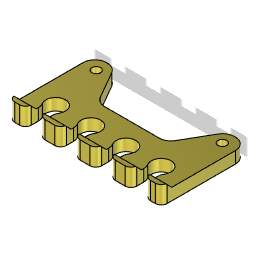
cable_holder (Autodesk Fusion 360 design; units mm, degrees)
Autodesk Fusion 360 part; units mm, degrees
note: some values were not read from the file. Set by a fixed rule: which sketch regions a step uses.
sketch "Sketch1" plane through (0, 0, 0) normal (0, 0, 1) x (1, 0, 0)
  line L0 (0, 0) -> (78, 0)
  line L1 (78, 0) -> (78, 24)
  line L2 (0, 24) -> (0, 0)
  line L3 (12, 12) -> (12, 24) construction
  line L4 (8.5, 15.5707) -> (15.5, 15.5707) construction
  line L5 (8.5, 15.5707) -> (8.5, 24)
  line L6 (15.5, 15.5707) -> (15.5, 24)
  arc A0 (8.5, 15.5707) -> (15.5, 15.5707) centre (12, 12) ccw
  line L7 (8.5, 24) -> (0, 24)
  line L8 (33.5, 15.5707) -> (33.5, 24)
  line L9 (26.5, 15.5707) -> (26.5, 24)
  arc A1 (26.5, 15.5707) -> (33.5, 15.5707) centre (30, 12) ccw
  line L10 (51.5, 15.5707) -> (51.5, 24)
  line L11 (44.5, 15.5707) -> (44.5, 24)
  arc A2 (44.5, 15.5707) -> (51.5, 15.5707) centre (48, 12) ccw
  line L12 (69.5, 15.5707) -> (69.5, 24)
  line L13 (62.5, 15.5707) -> (62.5, 24)
  arc A3 (62.5, 15.5707) -> (69.5, 15.5707) centre (66, 12) ccw
  line L14 (26.5, 24) -> (15.5, 24)
  line L15 (44.5, 24) -> (33.5, 24)
  line L16 (78, 24) -> (69.5, 24)
  line L17 (62.5, 24) -> (51.5, 24)
  dimension "d1" = 10
  dimension "d3" = 12
  dimension "d4" = 12
  dimension "d5" = 3.5
  dimension "d6" = 3.5
  dimension "d7" = 12
  dimension "d10" = 18
  dimension "d11" = 0
  dimension "d12" = 12
  constraint horizontal L0
  constraint vertical L1
  constraint horizontal L16
  constraint vertical L2
  constraint coincident L0.start L2.end
  constraint coincident L3.start A0.centre
  constraint perpendicular L3 L16
  constraint perpendicular L3 L4
  constraint coincident L5.end L16
  constraint perpendicular L4 L5
  constraint perpendicular L6 L16
  constraint collinear L7 L16
  constraint coincident L3.end L16
  constraint collinear L14 L16
  constraint collinear L15 L16
  constraint collinear L16 L17
  measures "d1" diameter of A0
  measures "d3" distance of L3.start L2
  measures "d4" distance of L3.start L0
  measures "d5" distance of L3 L4.end
  measures "d6" distance of L3 L4.start
  measures "d7" distance of L3.start L16
  measures "d12" distance of L1 A3.centre
  measures "d28" angle of L3.start
extrude "Extrude1" add sketch "Sketch1" along normal blind 9
sketch "Sketch2" plane through (0, 0, 0) normal (-1, 0, 0) x (0, -1, 0)
  line L0 (-24, 0) -> (0, 0)
  line L1 (0, 0) -> (0, 9)
  line L2 (0, 9) -> (-24, 9)
  line L3 (-24, 9) -> (-24, 0)
  line L4 (-24, 9) -> (-16.9844, 9) construction
  line L5 (-18.6, 6) -> (0, 6)
  line L6 (-24, 9) -> (0, 9)
  line L7 (0, 6) -> (0, 9)
  line L8 (-24, 9) -> (-21.6, 9)
  line L9 (-18.6, 6) -> (-21.6, 9)
  dimension "d17" = 3
  dimension "d34" = 45
  dimension "d35" = 2.4
  constraint horizontal L4
  constraint coincident L2.end L3.start
  constraint coincident L1 L5.end
  constraint perpendicular L1 L5
  constraint coincident L1.end L2.start
  constraint coincident L4 L8.end
  constraint perpendicular L3 L8
  measures "d17" distance of L2 L5
  measures "d34" angle of L6 L9
  measures "d35" distance of L2.end L8.end
extrude "Extrude2" cut sketch "Sketch2" against normal through all contours L1 L2 L5 L6 L7 L9
sketch "Sketch3" plane through (0, 0, 6) normal (0, 0, 1) x (-1, 0, 0)
  line L0 (-15.5, -18.6) -> (-15.5, -15.5707)
  arc A0 (-8.5, -15.5707) -> (-15.5, -15.5707) centre (-12, -12) ccw
  line L1 (-8.5, -15.5707) -> (-8.5, -18.6)
  line L2 (0, -18.6) -> (0, 0)
  line L3 (0, 0) -> (-78, 0)
  line L4 (-78, 0) -> (-78, -18.6)
  line L5 (-69.5, -18.6) -> (-69.5, -15.5707)
  arc A1 (-62.5, -15.5707) -> (-69.5, -15.5707) centre (-66, -12) ccw
  line L6 (-62.5, -15.5707) -> (-62.5, -18.6)
  line L7 (-51.5, -18.6) -> (-51.5, -15.5707)
  arc A2 (-44.5, -15.5707) -> (-51.5, -15.5707) centre (-48, -12) ccw
  line L8 (-44.5, -15.5707) -> (-44.5, -18.6)
  line L9 (-33.5, -18.6) -> (-33.5, -15.5707)
  arc A3 (-26.5, -15.5707) -> (-33.5, -15.5707) centre (-30, -12) ccw
  line L10 (-26.5, -15.5707) -> (-26.5, -18.6)
  line L11 (0, 0) -> (0, 20)
  line L12 (0, 20) -> (-10, 20)
  line L13 (-10, 20) -> (-21.547, 0)
  line L14 (-78, 0) -> (-78, 20)
  line L15 (-78, 20) -> (-68, 20)
  line L16 (-68, 20) -> (-56.453, 0)
  line L17 (0, 0) -> (-21.547, 0)
  line L18 (-56.453, 0) -> (-78, 0)
  line L19 (-8.5, -18.6) -> (0, -18.6)
  line L20 (-78, -18.6) -> (-69.5, -18.6)
  line L21 (-62.5, -18.6) -> (-51.5, -18.6)
  line L22 (-44.5, -18.6) -> (-33.5, -18.6)
  line L23 (-26.5, -18.6) -> (-15.5, -18.6)
  dimension "d25" = 20
  dimension "d26" = 10
  dimension "d27" = 10
  dimension "d28" = 60
  dimension "d29" = 60
  constraint coincident L2.end L3.start
  constraint perpendicular L3 L11
  constraint perpendicular L11 L12
  constraint coincident L3 L13.end
  constraint coincident L3.end L4.start
  constraint perpendicular L3 L14
  constraint perpendicular L14 L15
  constraint coincident L3 L16.end
  constraint collinear L12 L15
  measures "d25" distance of L2.end L11.end
  measures "d26" distance of L11.end L12.end
  measures "d27" distance of L14.end L15.end
  measures "d28" angle of L12 L13
  measures "d29" angle of L15 L16
extrude "Extrude3" add sketch "Sketch3" against normal up to surface (6 mm away) contours L3 L11 L12 L13 L17 | L3 L14 L15 L16 L18
sketch "Sketch4" plane through (0, 0, 6) normal (0, 0, 1) x (-1, 0, 0)
  line L0 (-15.5, -18.6) -> (-15.5, -15.5707)
  arc A0 (-8.5, -15.5707) -> (-15.5, -15.5707) centre (-12, -12) ccw
  line L1 (-8.5, -15.5707) -> (-8.5, -18.6)
  line L2 (-8.5, -18.6) -> (0, -18.6)
  line L3 (0, -18.6) -> (0, 20)
  line L4 (0, 20) -> (-10, 20)
  line L5 (-10, 20) -> (-21.547, 0)
  line L6 (-21.547, 0) -> (-56.453, 0)
  line L7 (-56.453, 0) -> (-68, 20)
  line L8 (-68, 20) -> (-78, 20)
  line L9 (-78, 20) -> (-78, -18.6)
  line L10 (-78, -18.6) -> (-69.5, -18.6)
  line L11 (-69.5, -18.6) -> (-69.5, -15.5707)
  arc A1 (-62.5, -15.5707) -> (-69.5, -15.5707) centre (-66, -12) ccw
  line L12 (-62.5, -15.5707) -> (-62.5, -18.6)
  line L13 (-62.5, -18.6) -> (-51.5, -18.6)
  line L14 (-51.5, -18.6) -> (-51.5, -15.5707)
  arc A2 (-44.5, -15.5707) -> (-51.5, -15.5707) centre (-48, -12) ccw
  line L15 (-44.5, -15.5707) -> (-44.5, -18.6)
  line L16 (-44.5, -18.6) -> (-33.5, -18.6)
  line L17 (-33.5, -18.6) -> (-33.5, -15.5707)
  arc A3 (-26.5, -15.5707) -> (-33.5, -15.5707) centre (-30, -12) ccw
  line L18 (-26.5, -15.5707) -> (-26.5, -18.6)
  line L19 (-26.5, -18.6) -> (-15.5, -18.6)
  circle A4 centre (-6.7321, 14) radius 2.25
  line L20 (0, 14) -> (-13.4641, 14) construction
  line L21 (-64.5359, 14) -> (-78, 14) construction
  circle A5 centre (-71.2679, 14) radius 2.25
  dimension "d36" = 4.5
  dimension "d37" = 6
  dimension "d38" = 4.5
  constraint coincident L3 L20.start
  constraint coincident L5 L20.end
  constraint perpendicular L3 L20
  constraint midpoint A4.centre L20
  constraint coincident L7 L21.start
  constraint coincident L9 L21.end
  constraint perpendicular L9 L21
  constraint midpoint L21 A5.centre
  constraint collinear L20 L21
  measures "d36" diameter of A4
  measures "d37" distance of L4 L20
  measures "d38" diameter of A5
extrude "Extrude5" cut sketch "Sketch4" against normal through all contours A4 | A5
fillet "Fillet1" radius 5.5 8 edges at (8.5, 15.5707, 3) (15.5, 15.5707, 3) (26.5, 15.5707, 3) (33.5, 15.5707, 3) (44.5, 15.5707, 3) (51.5, 15.5707, 3) (69.5, 15.5707, 3) (62.5, 15.5707, 3)
fillet "Fillet2" radius 3 10 edges at (69.5, 24, 4.5) (78, 24, 4.5) (62.5, 24, 4.5) (51.5, 24, 4.5) (44.5, 24, 4.5) (33.5, 24, 4.5) (26.5, 24, 4.5) (15.5, 24, 4.5) (8.5, 24, 4.5) (0, 24, 4.5)
fillet "Fillet3" radius 6 6 edges at (0, -20, 3) (10, -20, 3) (21.547, 0, 3) (56.453, 0, 3) (68, -20, 3) (78, -20, 3)
sketch "Sketch5" plane through (0, 0, 6) normal (0, 0, 1) x (-1, 0, 0)
  circle A0 centre (-6.7321, 14) radius 2.25
  circle A1 centre (-71.2679, 14) radius 2.25
  arc A2 (-72, 20) -> (-78, 14) centre (-72, 14) ccw
  line L0 (-78, 14) -> (-78, -18.6)
  line L1 (-78, -18.6) -> (-69.5, -18.6)
  line L2 (-69.5, -18.6) -> (-69.5, -17.4083)
  arc A3 (-69.5, -17.4083) -> (-70.2857, -14.5754) centre (-75, -17.4083) ccw
  arc A4 (-61.7143, -14.5754) -> (-70.2857, -14.5754) centre (-66, -12) ccw
  arc A5 (-61.7143, -14.5754) -> (-62.5, -17.4083) centre (-57, -17.4083) ccw
  line L3 (-62.5, -17.4083) -> (-62.5, -18.6)
  line L4 (-62.5, -18.6) -> (-51.5, -18.6)
  line L5 (-51.5, -18.6) -> (-51.5, -17.4083)
  arc A6 (-51.5, -17.4083) -> (-52.2857, -14.5754) centre (-57, -17.4083) ccw
  arc A7 (-43.7143, -14.5754) -> (-52.2857, -14.5754) centre (-48, -12) ccw
  arc A8 (-43.7143, -14.5754) -> (-44.5, -17.4083) centre (-39, -17.4083) ccw
  line L6 (-44.5, -17.4083) -> (-44.5, -18.6)
  line L7 (-44.5, -18.6) -> (-33.5, -18.6)
  line L8 (-33.5, -18.6) -> (-33.5, -17.4083)
  arc A9 (-33.5, -17.4083) -> (-34.2857, -14.5754) centre (-39, -17.4083) ccw
  arc A10 (-25.7143, -14.5754) -> (-34.2857, -14.5754) centre (-30, -12) ccw
  arc A11 (-25.7143, -14.5754) -> (-26.5, -17.4083) centre (-21, -17.4083) ccw
  line L9 (-26.5, -17.4083) -> (-26.5, -18.6)
  line L10 (-26.5, -18.6) -> (-15.5, -18.6)
  line L11 (-15.5, -18.6) -> (-15.5, -17.4083)
  arc A12 (-15.5, -17.4083) -> (-16.2857, -14.5754) centre (-21, -17.4083) ccw
  arc A13 (-7.7143, -14.5754) -> (-16.2857, -14.5754) centre (-12, -12) ccw
  arc A14 (-7.7143, -14.5754) -> (-8.5, -17.4083) centre (-3, -17.4083) ccw
  line L12 (-8.5, -17.4083) -> (-8.5, -18.6)
  line L13 (-8.5, -18.6) -> (0, -18.6)
  line L14 (0, -18.6) -> (0, 14)
  arc A15 (0, 14) -> (-6, 20) centre (-6, 14) ccw
  line L15 (-6, 20) -> (-6.5359, 20)
  arc A16 (-6.5359, 20) -> (-11.7321, 17) centre (-6.5359, 14) ccw
  line L16 (-11.7321, 17) -> (-19.815, 3)
  arc A17 (-25.0111, 0) -> (-19.815, 3) centre (-25.0111, 6) ccw
  line L17 (-25.0111, 0) -> (-52.9889, 0)
  arc A18 (-58.185, 3) -> (-52.9889, 0) centre (-52.9889, 6) ccw
  line L18 (-58.185, 3) -> (-66.2679, 17)
  arc A19 (-66.2679, 17) -> (-71.4641, 20) centre (-71.4641, 14) ccw
  line L19 (-71.4641, 20) -> (-72, 20)
  line L20 (109.7465, 0) -> (-156.5967, 0)
  line L21 (-156.5967, 0) -> (-156.5967, 57.2242)
  line L22 (-156.5967, 57.2242) -> (109.7465, 57.2242)
  line L23 (109.7465, 57.2242) -> (109.7465, 0)
  constraint horizontal L20
  constraint vertical L21
  constraint horizontal L22
  constraint vertical L23
  constraint collinear L17 L20
equation "d6 = d5"
equation "d27 = d26"
equation "d28 = 60 °"
equation "d29 = d28"
equation "d34 = 45 °"
